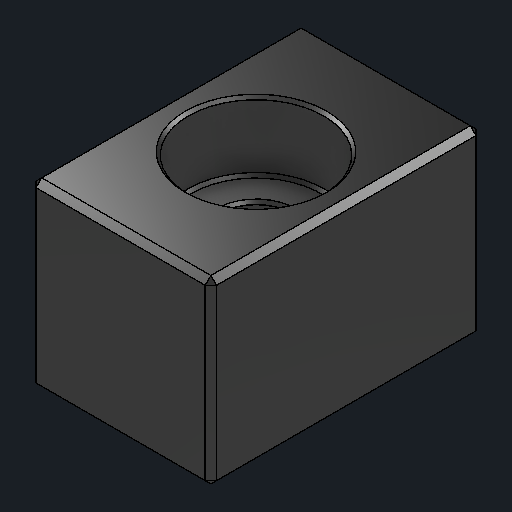
# Autodesk Inventor part: Fixture Stop
Saved by Autodesk Inventor 2026.2 (Build 302298000, 298)
## iProperties
Created: 2026-05-18
Part Number: Fixture Stop
Material: ABS Plastic
Document SubType Name: Modeling
Designer: JoshuaEah
Density: 1.06 g/cm^3
Appearance: Glossy - Black
Author: JoshuaEah
Autodesk Inventor part; units mm, degrees
ref_plane "YZ Plane" through (0, 0, 0) normal (1, 0, 0) x (0, 1, 0)
ref_plane "XZ Plane" through (0, 0, 0) normal (0, 1, 0) x (-1, 0, 0)
ref_plane "XY Plane" through (0, 0, 0) normal (0, 0, 1) x (1, 0, 0)
sketch "Sketch1" plane through (0, 0, 0) normal (0, 1, 0) x (-1, 0, 0)
  line L0 (0, 0) -> (-12.7, 0)
  line L1 (-12.7, 0) -> (-12.7, -19.05)
  line L2 (-12.7, -19.05) -> (0, -19.05)
  line L3 (0, -19.05) -> (0, 0)
  line L4 (-12.7, -9.525) -> (0, -9.525)
  circle A0 centre (-6.35, -9.525) radius 3.175 construction
  dimension "d0" = 12.7
  dimension "d1" = 19.05
  dimension "d2" = 6.35
  constraints: 10 end point, 3 midpoint, 2 parallel, 1 centre point, 1 coincident, 1 horizontal, 1 perpendicular
  measures "d0" distance of L2.end L1.end
  measures "d1" distance of L1.end L0.end
  measures "d2" diameter of A0
extrude "Extrusion1" add sketch "Sketch1" against normal blind 12.7
hole "Hole1" at (6.35, 0, -9.525) direction (0, -1, 0) diameter 5.1054 end through all counterbore diameter 9.525 counterbore depth 4.826 clearance for "Socket Head Cap Screw" size "#10" standard "Ansi Unified Screw Threads"
chamfer "Chamfer1" distance 0.4 angle 45 12 edges at (6.35, 0, -19.05) (12.7, 0, -9.525) (0, 0, -9.525) (6.35, 0, 0) (12.7, -6.35, 0) (12.7, -6.35, -19.05) (12.7, -12.7, -9.525) (6.35, -12.7, 0) (0, -6.35, 0) (0, -6.35, -19.05) (0, -12.7, -9.525) (6.35, -12.7, -19.05)
chamfer "Chamfer2" distance 0.2 angle 45 4 edges at (6.35, 0, -14.2875) (6.35, -12.7, -12.0777) (6.35, -4.826, -14.2875) (6.35, -4.826, -12.0777)
body "Solid1"
